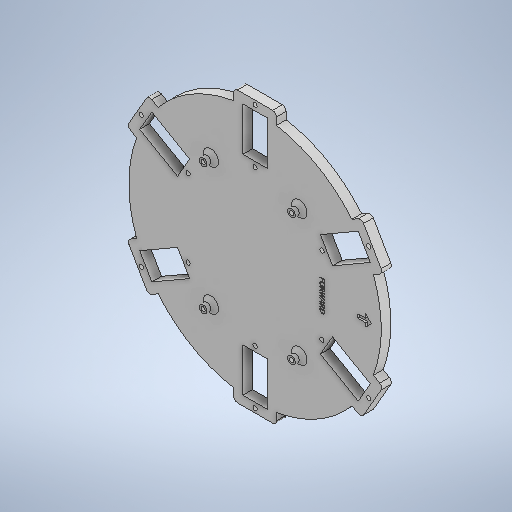
# Autodesk Inventor part: Base Plate v0.1
Saved by Autodesk Inventor 2025 (Build 290162000, 162)
## iProperties
Created: 2024-06-04
Part Number: Base Plate v0.1
Material: Generic
Document SubType Name: Modeling
Designer: sgols
Density: 1 g/cm^3
Appearance: Default
Author: sgols
Autodesk Inventor part; units mm, degrees
ref_plane "YZ Plane" through (0, 0, 0) normal (1, 0, 0) x (0, 1, 0)
ref_plane "XZ Plane" through (0, 0, 0) normal (0, 1, 0) x (-1, 0, 0)
ref_plane "XY Plane" through (0, 0, 0) normal (0, 0, 1) x (1, 0, 0)
sketch "Sketch1" plane through (0, 0, 0) normal (0, 0, 1) x (1, 0, 0)
  circle A0 centre (0, 0) radius 65
  dimension "d0" = 130
  constraints: 1 centre point, 1 coincident
  measures "d0" diameter of A0
extrude "Base plate" add sketch "Sketch1" along normal blind 5
sketch "Sketch2" plane through (0, 0, 5) normal (0, 0, 1) x (1, 0, 0)
  circle A0 centre (0, 0) radius 65 projected
  line L0 (-6.25, 65) -> (6.25, 65)
  line L1 (6.25, 65) -> (6.25, 42.5)
  line L2 (6.25, 42.5) -> (-6.25, 42.5)
  line L3 (-6.25, 42.5) -> (-6.25, 65)
  line L4 (11.05, 69.8) -> (-11.05, 69.8)
  line L5 (-11.05, 69.8) -> (-11.05, 37.7)
  line L6 (-11.05, 37.7) -> (11.05, 37.7)
  line L7 (11.05, 37.7) -> (11.05, 69.8)
  circle A1 centre (0, 67.65) radius 1.1
  line L8 (-11.05, 53.75) -> (11.05, 53.75) construction
  circle A2 centre (0, 39.85) radius 1.1
  point P0 (0, 65)
  point P1 (-11.05, 64.0539)
  point P2 (-6.25, 64.6988)
  point P3 (6.25, 64.6988)
  point P4 (11.05, 64.0539)
  dimension "d3" = 22.5
  dimension "d4" = 12.5
  dimension "d5" = 4.8
  dimension "d10" = 1.1
  dimension "d11" = 2.65
  constraints: 18 end point, 4 parallel, 3 midpoint, 2 centre point, 2 perpendicular, 2 vertical alignment, 1 horizontal, 1 symmetric about line, 6 other
  measures "d3" distance of L0.end L1.end
  measures "d4" distance of L0.start L0.end
  measures "d5" distance between parallel lines of L0 L4
  measures "d10" radius of A1
  measures "d11" distance of A1.centre point (0, 65)
extrude "Extrusion2" add sketch "Sketch2" against normal up to surface (5 mm away) contours A0 L1 L0 L3 L5 L4 L7 | A1
fillet "Fillet1" radius 2 2 edges at (-11.05, 69.8, 2.5) (11.05, 69.8, 2.5)
extrude "Screw Holes" cut sketch "Sketch2" against normal through all contours L1 L2 L3 A0 | A1 | A2
pattern_circular "Circular Pattern2" count 6 over 360 about axis through (0, 0, -10) along (0, 0, 1) of "Extrusion2", "Fillet1", "Screw Holes"
sketch "Sketch3" plane through (0, 0, 5) normal (0, 0, 1) x (1, 0, 0)
  line L0 (53, 0) -> (60, 0)
  line L1 (60, 0) -> (57, 3)
  line L2 (57, 3) -> (57, 1)
  line L3 (57, 1) -> (53, 1)
  line L4 (53, 1) -> (53, 0)
  arc A0 (60.9973, -22.4574) -> (60.9973, 22.4574) centre (0, 0) ccw projected
  line L5 (60, 0) -> (57, -3)
  line L6 (57, -3) -> (57, -1)
  line L7 (57, -1) -> (53, -1)
  line L8 (53, -1) -> (53, 0)
  line L9 (36, 7.996) -> (36, -7.996) construction
  line L10 (36, -7.996) -> (33.1609, -7.996) construction
  line L11 (33.1609, -7.996) -> (33.1609, 7.996) construction
  line L12 (33.1609, 7.996) -> (36, 7.996) construction
  line L13 (35.646, 6.2196) -> (35.646, 7.4011)
  line L14 (35.646, 7.4011) -> (34.9297, 7.4011)
  line L15 (34.9297, 7.4011) -> (34.9297, 6.269)
  line L16 (34.9297, 6.269) -> (34.6291, 6.269)
  line L17 (34.6291, 6.269) -> (34.6291, 7.4011)
  line L18 (34.6291, 7.4011) -> (33.4065, 7.4011)
  line L19 (33.4065, 7.4011) -> (33.4065, 7.7387)
  line L20 (33.4065, 7.7387) -> (35.9465, 7.7387)
  line L21 (35.9465, 7.7387) -> (35.9465, 6.2196)
  line L22 (35.9465, 6.2196) -> (35.646, 6.2196)
  spline S0 degree 2 poles (35.6563, 4.1201) (35.4875, 3.976) (34.9935, 3.8155) (34.6765, 3.8155) knots 0 0 0 1 2 2 2
  spline S1 degree 2 poles (34.6765, 3.8155) (34.3677, 3.8155) (33.8676, 3.9719) (33.6988, 4.1201) knots 0 0 0 1 2 2 2
  spline S2 degree 2 poles (33.6988, 4.1201) (33.5218, 4.2765) (33.353, 4.6903) (33.353, 4.9393) knots 0 0 0 1 2 2 2
  spline S3 degree 2 poles (33.353, 4.9393) (33.353, 5.1966) (33.5279, 5.6083) (33.6988, 5.7585) knots 0 0 0 1 2 2 2
  spline S4 degree 2 poles (33.6988, 5.7585) (33.8676, 5.9047) (34.3636, 6.0611) (34.6765, 6.0611) knots 0 0 0 1 2 2 2
  spline S5 degree 2 poles (34.6765, 6.0611) (34.9955, 6.0611) (35.4813, 5.9026) (35.6563, 5.7565) knots 0 0 0 1 2 2 2
  spline S6 degree 2 poles (35.6563, 5.7565) (35.825, 5.6083) (36, 5.1945) (36, 4.9393) knots 0 0 0 1 2 2 2
  spline S7 degree 2 poles (36, 4.9393) (36, 4.68) (35.8189, 4.2642) (35.6563, 4.1201) knots 0 0 0 1 2 2 2
  spline S8 degree 2 poles (34.6765, 4.1674) (34.9276, 4.1674) (35.3166, 4.2765) (35.4442, 4.3753) knots 0 0 0 1 2 2 2
  spline S9 degree 2 poles (35.4442, 4.3753) (35.576, 4.4762) (35.7077, 4.7602) (35.7077, 4.9373) knots 0 0 0 1 2 2 2
  spline S10 degree 2 poles (35.7077, 4.9373) (35.7077, 5.1204) (35.5801, 5.3963) (35.4442, 5.5012) knots 0 0 0 1 2 2 2
  spline S11 degree 2 poles (35.4442, 5.5012) (35.3146, 5.6021) (34.9235, 5.7091) (34.6765, 5.7091) knots 0 0 0 1 2 2 2
  spline S12 degree 2 poles (34.6765, 5.7091) (34.1763, 5.7091) (33.6453, 5.2892) (33.6453, 4.9373) knots 0 0 0 1 2 2 2
  spline S13 degree 2 poles (33.6453, 4.9373) (33.6453, 4.5853) (34.1763, 4.1674) (34.6765, 4.1674) knots 0 0 0 1 2 2 2
  line L23 (33.4065, 1.4792) -> (33.4065, 1.9177)
  line L24 (33.4065, 1.9177) -> (34.4171, 2.7204)
  line L25 (34.4171, 2.7204) -> (34.4171, 3.1074)
  line L26 (34.4171, 3.1074) -> (33.4065, 3.1074)
  line L27 (33.4065, 3.1074) -> (33.4065, 3.445)
  line L28 (33.4065, 3.445) -> (35.9465, 3.445)
  line L29 (35.9465, 3.445) -> (35.9465, 2.7904)
  spline S14 degree 2 poles (35.9465, 2.7904) (35.9465, 2.5722) (35.8991, 2.2779) (35.8127, 2.1441) knots 0 0 0 1 2 2 2
  spline S15 degree 2 poles (35.8127, 2.1441) (35.7262, 2.0103) (35.4566, 1.8559) (35.2569, 1.8559) knots 0 0 0 1 2 2 2
  spline S16 degree 2 poles (35.2569, 1.8559) (34.9791, 1.8559) (34.6024, 2.14) (34.5118, 2.3828) knots 0 0 0 1 2 2 2
  line L30 (34.5118, 2.3828) -> (33.4065, 1.4792)
  spline S17 degree 2 poles (35.2302, 2.2079) (35.3413, 2.2079) (35.5122, 2.2861) (35.5677, 2.3684) knots 0 0 0 1 2 2 2
  spline S18 degree 2 poles (35.5677, 2.3684) (35.6151, 2.4405) (35.6542, 2.6319) (35.6542, 2.7719) knots 0 0 0 1 2 2 2
  line L31 (35.6542, 2.7719) -> (35.6542, 3.1074)
  line L32 (35.6542, 3.1074) -> (34.6991, 3.1074)
  line L33 (34.6991, 3.1074) -> (34.6991, 2.811)
  spline S19 degree 2 poles (34.6991, 2.811) (34.6991, 2.6648) (34.7506, 2.4322) (34.8309, 2.352) knots 0 0 0 1 2 2 2
  spline S20 degree 2 poles (34.8309, 2.352) (34.9008, 2.2779) (35.0984, 2.2079) (35.2302, 2.2079) knots 0 0 0 1 2 2 2
  line L34 (35.9465, -1.5692) -> (33.4065, -0.9311)
  line L35 (33.4065, -0.9311) -> (33.4065, -0.5524)
  line L36 (33.4065, -0.5524) -> (35.5142, -0.0357)
  line L37 (35.5142, -0.0357) -> (33.4065, 0.4665)
  line L38 (33.4065, 0.4665) -> (33.4065, 0.8411)
  line L39 (33.4065, 0.8411) -> (35.9465, 1.4895)
  line L40 (35.9465, 1.4895) -> (35.9465, 1.1417)
  line L41 (35.9465, 1.1417) -> (33.8408, 0.6312)
  line L42 (33.8408, 0.6312) -> (35.9465, 0.1248)
  line L43 (35.9465, 0.1248) -> (35.9465, -0.2189)
  line L44 (35.9465, -0.2189) -> (33.8161, -0.7294)
  line L45 (33.8161, -0.7294) -> (35.9465, -1.2378)
  line L46 (35.9465, -1.2378) -> (35.9465, -1.5692)
  line L47 (33.4065, -1.598) -> (35.9465, -2.4543)
  line L48 (35.9465, -2.4543) -> (35.9465, -2.8701)
  line L49 (35.9465, -2.8701) -> (33.4065, -3.7263)
  line L50 (33.4065, -3.7263) -> (33.4065, -3.3702)
  line L51 (33.4065, -3.3702) -> (34.1166, -3.1397)
  line L52 (34.1166, -3.1397) -> (34.1166, -2.1702)
  line L53 (34.1166, -2.1702) -> (33.4065, -1.9397)
  line L54 (33.4065, -1.9397) -> (33.4065, -1.598)
  line L55 (34.4048, -3.0471) -> (35.6007, -2.6539)
  line L56 (35.6007, -2.6539) -> (34.4048, -2.2628)
  line L57 (34.4048, -2.2628) -> (34.4048, -3.0471)
  line L58 (33.4065, -5.9329) -> (33.4065, -5.4944)
  line L59 (33.4065, -5.4944) -> (34.4171, -4.6917)
  line L60 (34.4171, -4.6917) -> (34.4171, -4.3047)
  line L61 (34.4171, -4.3047) -> (33.4065, -4.3047)
  line L62 (33.4065, -4.3047) -> (33.4065, -3.9672)
  line L63 (33.4065, -3.9672) -> (35.9465, -3.9672)
  line L64 (35.9465, -3.9672) -> (35.9465, -4.6217)
  spline S21 degree 2 poles (35.9465, -4.6217) (35.9465, -4.8399) (35.8991, -5.1342) (35.8127, -5.268) knots 0 0 0 1 2 2 2
  spline S22 degree 2 poles (35.8127, -5.268) (35.7262, -5.4018) (35.4566, -5.5562) (35.2569, -5.5562) knots 0 0 0 1 2 2 2
  spline S23 degree 2 poles (35.2569, -5.5562) (34.9791, -5.5562) (34.6024, -5.2721) (34.5118, -5.0293) knots 0 0 0 1 2 2 2
  line L65 (34.5118, -5.0293) -> (33.4065, -5.9329)
  spline S24 degree 2 poles (35.2302, -5.2042) (35.3413, -5.2042) (35.5122, -5.126) (35.5677, -5.0437) knots 0 0 0 1 2 2 2
  spline S25 degree 2 poles (35.5677, -5.0437) (35.6151, -4.9716) (35.6542, -4.7802) (35.6542, -4.6402) knots 0 0 0 1 2 2 2
  line L66 (35.6542, -4.6402) -> (35.6542, -4.3047)
  line L67 (35.6542, -4.3047) -> (34.6991, -4.3047)
  line L68 (34.6991, -4.3047) -> (34.6991, -4.6011)
  spline S26 degree 2 poles (34.6991, -4.6011) (34.6991, -4.7473) (34.7506, -4.9799) (34.8309, -5.0601) knots 0 0 0 1 2 2 2
  spline S27 degree 2 poles (34.8309, -5.0601) (34.9008, -5.1342) (35.0984, -5.2042) (35.2302, -5.2042) knots 0 0 0 1 2 2 2
  spline S28 degree 2 poles (34.6744, -8.1374) (34.3266, -8.1374) (33.7667, -7.8554) (33.6103, -7.6187) knots 0 0 0 1 2 2 2
  spline S29 degree 2 poles (33.6103, -7.6187) (33.4888, -7.4252) (33.4065, -7.0279) (33.4065, -6.7192) knots 0 0 0 1 2 2 2
  line L69 (33.4065, -6.7192) -> (33.4065, -6.1346)
  line L70 (33.4065, -6.1346) -> (35.9465, -6.1346)
  line L71 (35.9465, -6.1346) -> (35.9465, -6.713)
  spline S30 degree 2 poles (35.9465, -6.713) (35.9465, -7.0711) (35.8394, -7.4787) (35.7448, -7.6228) knots 0 0 0 1 2 2 2
  spline S31 degree 2 poles (35.7448, -7.6228) (35.5822, -7.8677) (35.0449, -8.1374) (34.6744, -8.1374) knots 0 0 0 1 2 2 2
  spline S32 degree 2 poles (34.6785, -7.7854) (34.9708, -7.7854) (35.3846, -7.5919) (35.5019, -7.4005) knots 0 0 0 1 2 2 2
  spline S33 degree 2 poles (35.5019, -7.4005) (35.5822, -7.2646) (35.6542, -6.9579) (35.6542, -6.7295) knots 0 0 0 1 2 2 2
  line L72 (35.6542, -6.7295) -> (35.6542, -6.4722)
  line L73 (35.6542, -6.4722) -> (33.6988, -6.4722)
  line L74 (33.6988, -6.4722) -> (33.6988, -6.7295)
  spline S34 degree 2 poles (33.6988, -6.7295) (33.6988, -6.9538) (33.7708, -7.2934) (33.8676, -7.4313) knots 0 0 0 1 2 2 2
  spline S35 degree 2 poles (33.8676, -7.4313) (33.9869, -7.6084) (34.3821, -7.7854) (34.6785, -7.7854) knots 0 0 0 1 2 2 2
  point P0 (65, 0)
  point P1 (65, 0)
  point P2 (51, 0)
  point P3 (36, 0)
  point P4 (53, -0.5)
  dimension "d22" = 1
  dimension "d23" = 5
  dimension "d24" = 2
  dimension "d25" = 3
  dimension "d26" = 7
  dimension "d29" = 2
  constraints: 18 end point, 3 horizontal alignment, 3 perpendicular, 3 symmetric about line, 2 midpoint, 2 point on circle, 1 horizontal, 2 other
  measures "d22" distance of L3.end L0.start
  measures "d23" distance of point (65, 0) L0.end
  measures "d24" distance of L1.end L2.end
  measures "d25" horizontal distance of L2.end L0.end
  measures "d26" distance of L0.start L0.end
  measures "d29" distance of point (51, 0) L0.start
emboss "Emboss1" sketch "Sketch3" operation cut depth 1 direction (0, 0, -1)
sketch "Sketch4" plane through (0, 0, 5) normal (0, 0, 1) x (1, 0, 0)
  line L0 (22.8, 32.8) -> (-22.8, 32.8) construction
  line L1 (-22.8, 32.8) -> (-22.8, -32.8) construction
  line L2 (-22.8, -32.8) -> (22.8, -32.8) construction
  line L3 (22.8, -32.8) -> (22.8, 32.8) construction
  line L4 (22.8, 32.8) -> (-22.8, -32.8) construction
  line L5 (-22.8, 32.8) -> (22.8, -32.8) construction
  circle A0 centre (22.8, 32.8) radius 2
  circle A1 centre (-22.8, 32.8) radius 2
  circle A2 centre (-22.8, -32.8) radius 2
  circle A3 centre (22.8, -32.8) radius 2
  point P0 (0, 0)
  dimension "d32" = 65.6
  dimension "d33" = 45.6
  dimension "d41" = 4
  constraints: 12 end point, 4 centre point, 4 coincident, 3 equal radius, 2 midpoint, 2 parallel, 1 horizontal, 1 perpendicular
  measures "d32" distance of L0.end L1.end
  measures "d33" distance of L1.end L2.end
  measures "d41" diameter of A0
extrude "Perfboard Mounting Points" add sketch "Sketch4" along normal blind 4
fillet "Fillet2" radius 2 4 edges at (20.8, 32.8, 5) (20.8, -32.8, 5) (-24.8, -32.8, 5) (-24.8, 32.8, 5)
sketch "Sketch5" plane through (22.8, 32.8, 9) normal (0, 0, 1) x (1, 0, 0)
  circle A0 centre (0, 0) radius 2 projected
  circle A1 centre (-45.6, 0) radius 2 projected
  circle A2 centre (-45.6, -65.6) radius 2 projected
  circle A3 centre (0, -65.6) radius 2 projected
  point P0 (-22.8, -32.8)
  constraints: 4 coincident
hole "Hole2" at (22.8, 32.8, 9) at (-22.8, 32.8, 9) at (-22.8, -32.8, 9) at (22.8, -32.8, 9) direction (0, 0, -1) diameter 2.2 end through all
body "Solid1"
